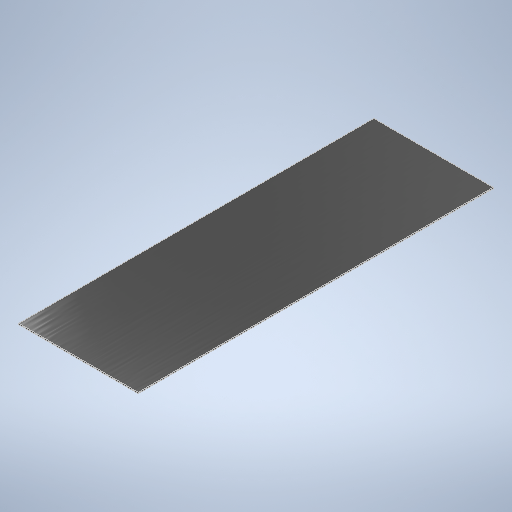
# Autodesk Inventor part: Shingle_With_Dimensions_13.25_x_39.375_Inches
Saved by Autodesk Inventor 2025.1 (Build 291241020, 241B)
## iProperties
Created: 2024-10-02
Part Number: Shingle_With_Dimensions_13.25_x_39.375_Inches
Material: Generic
Document SubType Name: Modeling
Designer: Tom
Density: 1 g/cm^3
Appearance: Dark Gray
Author: Tom
Autodesk Inventor part; units mm, degrees
ref_plane "YZ Plane" through (0, 0, 0) normal (1, 0, 0) x (0, 1, 0)
ref_plane "XZ Plane" through (0, 0, 0) normal (0, 1, 0) x (-1, 0, 0)
ref_plane "XY Plane" through (0, 0, 0) normal (0, 0, 1) x (1, 0, 0)
sketch "Sketch1" plane through (0, 0, 0) normal (0, 1, 0) x (-1, 0, 0)
  line L0 (0, 0) -> (336.55, 0)
  line L1 (336.55, 0) -> (336.55, -1000.125)
  line L2 (336.55, -1000.125) -> (0, -1000.125)
  line L3 (0, -1000.125) -> (0, 0)
  dimension "d0" = 336.55
  dimension "d1" = 1000.125
  constraints: 8 end point, 2 parallel, 1 horizontal, 1 perpendicular
  measures "d0" distance of L0.start L0.end
  measures "d1" distance of L2.end L0.start
extrude "Extrusion1" add sketch "Sketch1" along normal blind 3.175
body "Solid1"
